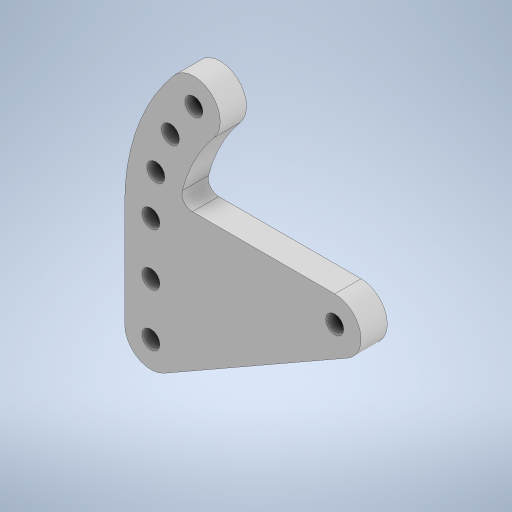
# Autodesk Inventor part: side_part
Saved by Autodesk Inventor 2024.3 (Build 283343010, 343A)
## iProperties
Created: 2025-07-19
Part Number: side_part
Material: 一般
Document SubType Name: Modeling
Designer: hikou
Density: 1 g/cm^3
Appearance: 既定
Author: hikou
Autodesk Inventor part; units mm, degrees
ref_plane "YZ Plane" through (0, 0, 0) normal (1, 0, 0) x (0, 1, 0)
ref_plane "XZ Plane" through (0, 0, 0) normal (0, 1, 0) x (-1, 0, 0)
ref_plane "XY Plane" through (0, 0, 0) normal (0, 0, 1) x (1, 0, 0)
sketch "スケッチ1" plane through (0, 0, 0) normal (0, 0, 1) x (1, 0, 0)
  circle A0 centre (0, 0) radius 40
  line L0 (0, 0) -> (0, 40)
  line L1 (-40, 0) -> (0, 0)
  dimension "d0" = 80
  constraints: 4 end point, 2 point on circle, 1 centre point, 1 coincident, 1 perpendicular
  measures "d0" diameter of A0
extrude "押し出し1" add sketch "スケッチ1" along normal mid plane 5 contours L0 L1 A0 picked at (-23.4047, 12.51)
sketch "スケッチ2" plane through (0, 0, 2.5) normal (0, 0, 1) x (1, 0, 0)
  line L0 (0, 0) -> (0, 40) projected
  arc A0 (0, 40) -> (-40, 0) centre (0, 0) ccw projected
  line L1 (-40, 0) -> (0, 0) projected
  line L2 (-40, 0) -> (0, 0)
  line L3 (0, 0) -> (0, -5)
  line L4 (0, -5) -> (-40, -5)
  line L5 (-40, -5) -> (-40, 0)
  line L6 (0, -5) -> (5, -5)
  line L7 (5, -5) -> (5, 5)
  line L8 (5, 5) -> (0, 5)
  line L9 (0, 5) -> (0, -5)
  dimension "d3" = 5
  dimension "d4" = 5
  dimension "d5" = 10
  constraints: 16 end point, 4 parallel, 2 horizontal, 2 perpendicular
  measures "d3" distance of L2.end L3.end
  measures "d4" distance of L8.end L7.end
  measures "d5" distance of L7.end L6.end
extrude "押し出し2" add sketch "スケッチ2" against normal blind 5 contours L3 L4 L5 L1 | L0 L8 L7 L6 L3
sketch "スケッチ3" plane through (0, 0, 2.5) normal (0, 0, 1) x (1, 0, 0)
  circle A0 centre (0, 0) radius 35
  point P0 (-35, 0)
  point P1 (-34.0566, 8.0716)
  point P2 (-31.2771, 15.708)
  point P3 (-26.8116, 22.4976)
  dimension "d8" = 70
  dimension "d11" = 40
  constraints: 2 coincident, 1 horizontal alignment, 6 other
hole "穴1" at (0, 0, 2.5) at (-35, 0, 2.5) at (-34.0566, 8.0716, 2.5) at (-31.2771, 15.708, 2.5) at (-26.8116, 22.4976, 2.5) direction (0, 0, -1) diameter 3.4 end through all
sketch "スケッチ4" plane through (0, 0, 2.5) normal (0, 0, 1) x (1, 0, 0)
  arc A0 (-1.7, 0) -> (-1.7, 0) centre (0, 0) ccw projected
  circle A1 centre (0, 0) radius 30
  circle A2 centre (-26.8116, 22.4976) radius 1.7 projected
  circle A3 centre (-31.2771, 15.708) radius 1.7 projected
  circle A4 centre (-34.0566, 8.0716) radius 1.7 projected
  circle A5 centre (-35, 0) radius 1.7 projected
  circle A6 centre (0, 0) radius 1.7 projected
  line L0 (0, 5) -> (0, 40) projected
  arc A7 (0, 40) -> (-40, 0) centre (0, 0) ccw projected
  line L1 (-40, 0) -> (-40, -5) projected
  line L2 (-40, -5) -> (5, -5) projected
  line L3 (5, -5) -> (5, 5) projected
  line L4 (5, 5) -> (0, 5) projected
  line L5 (0, 0) -> (-30.6418, 25.7115)
  line L6 (-30.6418, 25.7115) -> (-22.9813, 19.2836)
  line L7 (-22.9813, 19.2836) -> (-19.7674, 23.1139)
  line L8 (-19.7674, 23.1139) -> (-27.4278, 29.5417)
  line L9 (-27.4278, 29.5417) -> (-30.6418, 25.7115)
  line L10 (0, 5) -> (-29.5804, 5)
  point P0 (-27.1875, 29.3401)
  dimension "d20" = 60
  dimension "d21" = 40
  dimension "d22" = 5
  constraints: 12 end point, 3 point on circle, 2 parallel, 1 centre point, 1 coincident, 1 horizontal, 1 perpendicular, 1 point on line
  measures "d20" diameter of A1
  measures "d21" angle of L2 L5
  measures "d22" distance of L7.end L6.end
extrude "押し出し3" cut sketch "スケッチ4" against normal blind 55 contours L10 A1 L5 | L5 A1 L0 L10 | L7 L8 A7 L0 A1
sketch "スケッチ7" plane through (0, 0, 2.5) normal (0, 0, 1) x (1, 0, 0)
  line L0 (-40, -5) -> (5, -5) projected
  line L1 (-40, -5) -> (-30, -5)
  line L2 (-30, -5) -> (-30, -25)
  line L3 (-30, -25) -> (-40, -25)
  line L4 (-40, -25) -> (-40, -5)
  line L5 (-30, -25) -> (5, -5)
  point P0 (0, 0)
  dimension "d40" = 10
  dimension "d41" = 20
  constraints: 10 end point, 2 parallel, 1 horizontal, 1 perpendicular
  measures "d40" distance of L2.end L3.end
  measures "d41" distance of L1.end L2.end
extrude "押し出し5" add sketch "スケッチ7" against normal blind 5
sketch "スケッチ8" plane through (0, 0, 2.5) normal (0, 0, 1) x (1, 0, 0)
  line L0 (-40, 0) -> (-40, -25) projected
  line L1 (-40, -25) -> (-30, -25) projected
  point P0 (0, 0)
  point P1 (-35, -10)
  point P2 (-35, -20)
  dimension "d44" = 5
  dimension "d45" = 5
  dimension "d46" = 10
  dimension "d47" = 5
  measures "d44" distance from line of L0 point (-35, -20)
  measures "d45" distance from line of L1 point (-35, -20)
  measures "d46" distance of point (-35, -20) point (-35, -10)
  measures "d47" distance from line of L0 point (-35, -10)
hole "穴3" at (-35, -20, 2.5) at (-35, -10, 2.5) direction (0, 0, -1) diameter 3.4 end through all
sketch "スケッチ9" plane through (0, 0, 2.5) normal (0, 0, 1) x (1, 0, 0)
  circle A0 centre (0, 0) radius 1.7 projected
  circle A1 centre (0, 0) radius 5
  line L0 (-29.5804, 5) -> (5, 5) projected
  circle A2 centre (-35, -20) radius 1.7 projected
  circle A3 centre (-35, -20) radius 5
  line L1 (-40, -25) -> (-40, 0) projected
  line L2 (-35, -20) -> (0, 0) construction
  line L3 (-32.5193, -24.3412) -> (2.4807, -4.3412)
  line L4 (-2.4807, 4.3412) -> (-37.4807, -15.6588)
  arc A4 (-37.4807, -15.6588) -> (-32.5193, -24.3412) centre (-35, -20) ccw
  arc A5 (2.4807, -4.3412) -> (-2.4807, 4.3412) centre (0, 0) ccw
  circle A6 centre (-35, -10) radius 1.7 projected
  circle A7 centre (-35, -20) radius 1.7 projected
  line L5 (-19.7674, 23.1139) -> (-27.1875, 29.3401) projected
  arc A8 (-27.1875, 29.3401) -> (-40, 0) centre (0, 0) ccw projected
  line L6 (-40, 0) -> (-40, -25) projected
  line L7 (-40, -25) -> (-30, -25) projected
  line L8 (-30, -25) -> (5, -5) projected
  line L9 (5, -5) -> (5, 5) projected
  line L10 (5, 5) -> (-29.5804, 5) projected
  arc A9 (-22.9813, 19.2836) -> (-29.5804, 5) centre (0, 0) ccw projected
  line L11 (-22.9813, 19.2836) -> (-19.7674, 23.1139) projected
  circle A10 centre (-26.8116, 22.4976) radius 1.7 projected
  circle A11 centre (-31.2771, 15.708) radius 1.7 projected
  circle A12 centre (-34.0566, 8.0716) radius 1.7 projected
  circle A13 centre (-35, 0) radius 1.7 projected
  circle A14 centre (0, 0) radius 1.7 projected
  circle A15 centre (-26.8116, 22.4976) radius 5
  point P0 (-17.5, -10)
  point P1 (5, 0)
  point P2 (2.4807, -4.3412)
  point P3 (-35, -25)
  point P4 (0, 5)
  point P5 (-40, -20)
  point P6 (-22.9813, 19.2836)
  point P7 (-23.5976, 26.3278)
  point P8 (-30.6418, 25.7115)
  constraints: 8 end point, 7 tangent, 5 centre point, 4 point on circle, 3 coincident, 1 concentric, 1 midpoint, 1 parallel
extrude "押し出し6" cut sketch "スケッチ9" against normal blind 5 contours A1 L9 L8 L7 A3 L3 | L0 L9 A1 | A3 L7 L1 | A15 L5 L11 | A8 L5 A15
fillet "フィレット1" radius 2 1 edges at (-29.5804, 5, 0)
equation "\"d45\" = d44"
equation "\"d47\" = d44"
